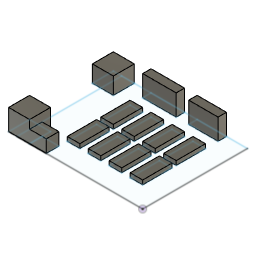
cafe v1 (Autodesk Fusion 360 design; units mm, degrees)
Autodesk Fusion 360 part; units mm, degrees
sketch "Sketch1" plane through (0, 0, 0) normal (0, 0, 1) x (1, 0, 0)
  line L0 (0, 0) -> (-150, 0)
  line L1 (-150, 0) -> (-150, 125)
  line L2 (-150, 125) -> (0, 125)
  line L3 (0, 125) -> (0, 0)
  line L4 (-160, 25) -> (-135, 25)
  line L5 (-135, 25) -> (-135, 0)
  line L6 (-135, 0) -> (-160, 0)
  line L7 (-160, 0) -> (-160, 25)
  line L8 (-160, 125) -> (-135, 125)
  line L9 (-135, 125) -> (-135, 100)
  line L10 (-135, 100) -> (-160, 100)
  line L11 (-160, 100) -> (-160, 125)
  line L12 (-135, 15) -> (-115, 15)
  line L13 (-115, 15) -> (-115, 0)
  line L14 (-115, 0) -> (-135, 0)
  line L15 (-135, 0) -> (-135, 15)
  line L16 (-115, 125) -> (-75, 125)
  line L17 (-75, 125) -> (-75, 115)
  line L18 (-75, 115) -> (-115, 115)
  line L19 (-115, 115) -> (-115, 125)
  line L20 (-60, 125) -> (-25, 125)
  line L21 (-25, 125) -> (-25, 115)
  line L22 (-25, 115) -> (-60, 115)
  line L23 (-60, 115) -> (-60, 125)
  line L24 (-115, 100) -> (-100, 100)
  line L25 (-100, 100) -> (-100, 65)
  line L26 (-100, 65) -> (-115, 65)
  line L27 (-115, 65) -> (-115, 100)
  line L28 (-115, 60) -> (-100, 60)
  line L29 (-100, 60) -> (-100, 25)
  line L30 (-100, 25) -> (-115, 25)
  line L31 (-115, 25) -> (-115, 60)
  line L32 (-90, 100) -> (-75, 100)
  line L33 (-75, 100) -> (-75, 65)
  line L34 (-75, 65) -> (-90, 65)
  line L35 (-90, 65) -> (-90, 100)
  line L36 (-65, 100) -> (-50, 100)
  line L37 (-50, 100) -> (-50, 65)
  line L38 (-50, 65) -> (-65, 65)
  line L39 (-65, 65) -> (-65, 100)
  line L40 (-40, 100) -> (-25, 100)
  line L41 (-25, 100) -> (-25, 65)
  line L42 (-25, 65) -> (-40, 65)
  line L43 (-40, 65) -> (-40, 100)
  line L44 (-90, 60) -> (-75, 60)
  line L45 (-75, 60) -> (-75, 25)
  line L46 (-75, 25) -> (-90, 25)
  line L47 (-90, 25) -> (-90, 60)
  line L48 (-65, 60) -> (-50, 60)
  line L49 (-50, 60) -> (-50, 25)
  line L50 (-50, 25) -> (-65, 25)
  line L51 (-65, 25) -> (-65, 60)
  line L52 (-40, 60) -> (-25, 60)
  line L53 (-25, 60) -> (-25, 25)
  line L54 (-25, 25) -> (-40, 25)
  line L55 (-40, 25) -> (-40, 60)
  constraint horizontal L0
  constraint vertical L1
  constraint horizontal L2
  constraint vertical L3
  constraint coincident L0.start L3.end
  constraint horizontal L4
  constraint vertical L5
  constraint horizontal L6
  constraint vertical L7
  constraint coincident L0 L5.end
  constraint horizontal L8
  constraint vertical L9
  constraint horizontal L10
  constraint vertical L11
  constraint horizontal L12
  constraint vertical L13
  constraint horizontal L14
  constraint vertical L15
  constraint coincident L0 L13.end
  constraint coincident L5 L12.start
  constraint horizontal L16
  constraint vertical L17
  constraint horizontal L18
  constraint vertical L19
  constraint coincident L2 L16.start
  constraint horizontal L20
  constraint vertical L21
  constraint horizontal L22
  constraint vertical L23
  constraint coincident L2 L20.start
  constraint horizontal L24
  constraint vertical L25
  constraint horizontal L26
  constraint vertical L27
  constraint horizontal L28
  constraint vertical L29
  constraint horizontal L30
  constraint vertical L31
  constraint horizontal L32
  constraint vertical L33
  constraint horizontal L34
  constraint vertical L35
  constraint horizontal L36
  constraint vertical L37
  constraint horizontal L38
  constraint vertical L39
  constraint horizontal L40
  constraint vertical L41
  constraint horizontal L42
  constraint vertical L43
  constraint horizontal L44
  constraint vertical L45
  constraint horizontal L46
  constraint vertical L47
  constraint horizontal L48
  constraint vertical L49
  constraint horizontal L50
  constraint vertical L51
  constraint horizontal L52
  constraint vertical L53
  constraint horizontal L54
  constraint vertical L55
extrude "Extrude1" add sketch "Sketch1" along normal blind 5 contours L24 L25 L26 L27 | L28 L29 L30 L31 | L32 L33 L34 L35 | L36 L37 L38 L39 | L40 L41 L42 L43 | L44 L45 L46 L47 | L48 L49 L50 L51 | L52 L53 L54 L55 makes body 1 at (-60, 88.3333, 0) makes body 2 at (-110, 88.3333, 0) makes body 3 at (-85, 88.3333, 0) makes body 4 at (-35, 48.3333, 0) makes body 5 at (-60, 48.3333, 0) makes body 6 at (-110, 48.3333, 0) makes body 7 at (-85, 48.3333, 0) makes body 8 at (-35, 88.3333, 0)
extrude "Extrude2" add sketch "Sketch1" along normal blind 25 separate body contours L2 L20 L21 L22 L23 | L2 L16 L17 L18 L19 makes body 9 at (-88.3333, 115, 8.3333) makes body 10 at (-36.6667, 115, 8.3333)
extrude "Extrude3" add sketch "Sketch1" along normal blind 25 separate body contours L0 L1 L4 L5 L6 L15 | L1 L4 L6 L7 makes body 11
extrude "Extrude4" add sketch "Sketch1" along normal blind 15 contours L0 L5 L12 L13 L14 L15 bodies 11
extrude "Extrude5" add sketch "Sketch1" along normal blind 20 separate body contours L1 L8 L10 L11 | L1 L2 L8 L9 L10 makes body 12
